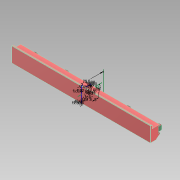
# Autodesk Inventor part: RailVCoverST
Saved by Autodesk Inventor 2021 (Build 250183000, 183)
## iProperties
Created: 2021-03-17
Part Number: RailVCoverST
Material: 一般
Document SubType Name: Modeling
Designer: kumagai
Density: 1 g/cm^3
Appearance: 滑らか - 濃い海緑
Length: 185.000 mm
PrinterOffset: 0.000 mm
StraightLength: 215.000 mm
RailWidth: 38.000 mm
OuterWall: 2.000 mm
InnerWall: 2.400 mm
InsideWidth: 18.600 mm
RailHeight: 8.400 mm
RailDepth: 3.200 mm
ConnectorLength: 15.000 mm
JointMW1: 13.000 mm
JointMW2: 9.400 mm
JointMH: 9.000 mm
JointFW1: 13.300 mm
JointFW2: 9.600 mm
JointFH: 9.500 mm
DoubleWidth: 60.000 mm
ViaductHeight: 66.000 mm
SupportGap: 0.200 mm
SupportRib: 0.500 mm
FixInterval: 41.250 mm
FixNum: 5.000 ul
Author: kumagai
Autodesk Inventor part; units mm, degrees
ref_plane "YZ Plane" through (0, 0, 0) normal (1, 0, 0) x (0, 1, 0)
ref_plane "XZ Plane" through (0, 0, 0) normal (0, 1, 0) x (-1, 0, 0)
ref_plane "XY Plane" through (0, 0, 0) normal (0, 0, 1) x (1, 0, 0)
sketch "スケッチ1" plane through (0, 0, 0) normal (1, 0, 0) x (0, 1, 0)
  line L0 (-5.88, 0) -> (5.88, 0) projected
  line L1 (0, 22.8) -> (0, -3.8) projected
  line L2 (1, 9.3) -> (1, 17)
  line L3 (1, 17) -> (4.2, 17)
  line L4 (4.2, 17) -> (4.2, 19)
  line L5 (4.2, 19) -> (-4.2, 19)
  line L6 (-4.2, 19) -> (-4.2, 17)
  line L7 (-4.2, 17) -> (-1, 17)
  line L8 (-1, 17) -> (-1, 9.3)
  line L9 (-1, 9.3) -> (-4.2, 9.3)
  line L10 (-4.2, 9.3) -> (-4.2, 6.9)
  line L11 (-4.2, 6.9) -> (-1, 6.9)
  line L12 (-1, 6.9) -> (-1, 0)
  line L13 (1, 9.3) -> (4.2, 9.3)
  line L14 (4.2, 9.3) -> (4.2, 6.9)
  line L15 (4.2, 6.9) -> (1, 6.9)
  line L16 (1, 6.9) -> (1, 0)
  line L17 (-4.2, 19) -> (-4.2, 17)
  line L18 (4.2, 17) -> (3.7, 17)
  point P0 (0, 0)
  dimension "d0" = 19
  dimension "d1" = 8.4
  dimension "d2" = 3.2
  dimension "d3" = 2
  dimension "d4" = 2.4
  dimension "d5" = 9.3
  constraints: 34 end point, 13 point on line, 9 perpendicular, 2 collinear, 1 horizontal, 1 vertical, 2 other
  measures "d0" distance between parallel lines of L5 L0
  measures "d1" distance between parallel lines of L6 L4
  measures "d2" distance between parallel lines of L16 L14
  measures "d3" distance between parallel lines of L5 L3
  measures "d4" distance between parallel lines of L15 L13
  measures "d5" distance between parallel lines of L0 L13
sketch "スケッチ2" plane through (0, 0, 0) normal (1, 0, 0) x (0, 1, 0)
  line L0 (10, 29.5) -> (-10, 29.5)
  line L1 (-10, 29.5) -> (-10, 22.3641)
  line L2 (10, 27.5) -> (10, 29.5)
  line L3 (-4.299, 19.1) -> (-4.299, 17)
  line L4 (4.6, 17.1) -> (5.22, 17.1)
  line L5 (4.6, 26.3) -> (3.5931, 27.5)
  line L6 (5.22, 17.1) -> (5.62, 17.5)
  line L7 (5.62, 17.5) -> (5.62, 27.5)
  line L8 (0, 34.06) -> (0, 2.14) projected
  line L9 (-14, 0) -> (14, 0) projected
  line L10 (4.2, 17) -> (4.2, 19) projected
  line L11 (-4.299, 19.1) -> (-4.299, 17)
  line L12 (-5.299, 24.1048) -> (-5.299, 26.3)
  line L13 (-5.299, 26.3) -> (-6.3059, 27.5)
  line L14 (-9.4, 23.2048) -> (-5.299, 23.2048)
  line L15 (-5.299, 23.2048) -> (-5.299, 20)
  line L16 (-9.4, 27.5) -> (-6.3059, 27.5)
  line L17 (-4.299, 27.5) -> (3.5931, 27.5)
  line L18 (5.62, 27.5) -> (10, 27.5)
  line L19 (-5.299, 20) -> (-6.7109, 20)
  line L20 (-10, 22.3641) -> (-5.499, 17)
  line L21 (3.5931, 20.4) -> (-4.299, 20.4)
  line L22 (-9.4, 27.5) -> (-9.4, 24.1048)
  line L23 (-9.4, 23.2048) -> (-6.7109, 20)
  line L24 (-5.299, 24.1048) -> (-9.4, 24.1048)
  line L25 (-4.299, 27.5) -> (-4.299, 20.4)
  line L26 (-4.299, 24.3119) -> (-4.299, 20.4)
  line L27 (4.6, 26.3) -> (4.6, 21.4069)
  line L28 (4.6, 21.4069) -> (3.5931, 20.4)
  line L29 (-4.2, 19) -> (-4.2, 17) projected
  line L30 (4.2, 19) -> (-4.2, 19) projected
  line L31 (-4.299, 17) -> (-5.499, 17)
  line L32 (-4.299, 19.1) -> (4.3, 19.1)
  line L33 (4.3, 19.1) -> (4.6, 18.5804)
  line L34 (4.6, 18.5804) -> (4.6, 17.1)
  line L35 (-1, 9.3) -> (-4.2, 9.3) projected
  line L36 (-4.2, 9.3) -> (-4.2, 6.9) projected
  line L37 (-4.2, 6.9) -> (-1, 6.9) projected
  line L38 (-4.299, 17) -> (-4.299, 6.7)
  line L39 (-4.299, 6.7) -> (-9.299, 6.7)
  line L40 (-9.299, 6.7) -> (-10, 7.5354)
  line L41 (-10, 16.6215) -> (-7.5247, 13.6715)
  line L42 (-7.5247, 13.6715) -> (-6.299, 14.7)
  line L43 (-6.299, 14.7) -> (-10, 19.1107)
  line L44 (-10, 7.5354) -> (-10, 16.6215)
  line L45 (-10, 19.1107) -> (-10, 22.3641)
  point P0 (-3.7, 17)
  point P1 (-3.2, 19)
  point P2 (3.7, 17)
  point P3 (0, 20.4)
  dimension "d63" = 29.5
  dimension "d71" = 2
  dimension "d72" = 40
  dimension "d73" = 1.2
  dimension "d93" = 0.2
  dimension "d109" = 40
  dimension "d110" = 2
  dimension "d113" = 1
  dimension "d114" = 0.6
  dimension "d115" = 0.9
  dimension "d117" = 1
  dimension "d128" = 1.02
  dimension "d129" = 45
  dimension "d130" = 0.4
  dimension "d141" = 0.099
  dimension "d142" = 5.8
  dimension "d143" = 5.8
  dimension "d144" = 3
  dimension "d145" = 0.1
  dimension "d146" = 1.3
  dimension "d147" = 30
  dimension "d148" = 0.1
  dimension "d149" = 0.4
  dimension "d150" = 0.1
  dimension "d151" = 45
  dimension "d152" = 0.2
  dimension "d153" = 5
  dimension "d156" = 1.6
  dimension "d157" = 2
  dimension "d158" = 8
  constraints: 77 end point, 16 perpendicular, 9 parallel, 6 horizontal, 5 collinear, 5 vertical, 3 point on line, 1 horizontal alignment, 1 vertical alignment
  measures "d63" distance between parallel lines of L0 L9
  measures "d71" distance between parallel lines of L0 L16
  measures "d72" angle of L12 L13
  measures "d73" distance from line of L12.end L16
  measures "d93" horizontal distance of L20.end L15.end
  measures "d109" angle of L8 L20
  measures "d110" distance between parallel lines of L0 L18
  measures "d113" distance between parallel lines of L20 L23
  measures "d114" distance between parallel lines of L1 L22
  measures "d115" distance between parallel lines of L24 L14
  measures "d117" distance between parallel lines of L12 L26
  measures "d128" distance between parallel lines of L7 L27
  measures "d129" angle of L4 L6
  measures "d130" distance from line of L4 L6.end
  measures "d141" distance between parallel lines of L3 L29
  measures "d142" distance between parallel lines of L1 L29
  measures "d143" distance between parallel lines of L2 L10
  measures "d144" distance between parallel lines of L31 L19
  measures "d145" distance between parallel lines of L30 L32
  measures "d146" distance between parallel lines of L21 L32
  measures "d147" angle of L10 L33
  measures "d148" distance from line of L10 L32.end
  measures "d149" distance between parallel lines of L10 L34
  measures "d150" distance from line of L4 L10.start
  measures "d151" angle of L27 L28
  measures "d152" distance between parallel lines of L39 L37
  measures "d153" distance from line of L39.end L38
  measures "d156" distance between parallel lines of L41 L43
  measures "d157" distance from line of L38 L42.end
  measures "d158" distance from line of L39 L42.end
extrude "押し出し3" [suppressed]
extrude "押し出し4" add sketch "スケッチ2" along normal mid plane 185 contours L2 L18 L7 L6 L4 L34 L33 L32 L8 L21 L28 L27 L5 L17 L0 | L8 L17 L25 L21 L32 L3 L31 L20 L1 L0
chamfer "面取り1" distance 0.4 angle 45 2 edges at (0, 10, 29.5) (0, 10, 27.5)
sketch "スケッチ3" plane through (92.5, 0, 0) normal (1, 0, 0) x (0, 0, -1)
  line L0 (-27.9, 10) -> (-27.5, 9.6) projected
  line L1 (-27.9, 10) -> (-29.1, 10) projected
  line L2 (-29.5, 9.6) -> (-29.1, 10) projected
  line L3 (-29.5, 9.6) -> (-29.5, -10) projected
  line L4 (-29.5, -10) -> (-22.3641, -10) projected
  line L5 (-22.3641, -10) -> (-17, -5.499) projected
  line L6 (-17, -4.299) -> (-19.1, -4.299) projected
  line L7 (-17.1, 4.6) -> (-17.1, 5.22) projected
  line L8 (-17.1, 5.22) -> (-17.5, 5.62) projected
  line L9 (-17.5, 5.62) -> (-27.5, 5.62) projected
  line L10 (-27.5, 5.62) -> (-27.5, 9.6) projected
  line L11 (-27.5, -9.4) -> (-27.5, -6.3059) projected
  line L12 (-27.5, -6.3059) -> (-26.3, -5.299) projected
  line L13 (-26.3, -5.299) -> (-24.1048, -5.299) projected
  line L14 (-24.1048, -5.299) -> (-24.1048, -9.4) projected
  line L15 (-24.1048, -9.4) -> (-27.5, -9.4) projected
  line L16 (-23.2048, -9.4) -> (-23.2048, -5.299) projected
  line L17 (-23.2048, -5.299) -> (-20, -5.299) projected
  line L18 (-20, -5.299) -> (-20, -6.7109) projected
  line L19 (-20, -6.7109) -> (-23.2048, -9.4) projected
  line L20 (-26.3, 4.6) -> (-21.4069, 4.6) projected
  line L21 (-21.4069, 4.6) -> (-20.4, 3.5931) projected
  line L22 (-20.4, 3.5931) -> (-20.4, -4.299) projected
  line L23 (-20.4, -4.299) -> (-27.5, -4.299) projected
  line L24 (-27.5, -4.299) -> (-27.5, 3.5931) projected
  line L25 (-27.5, 3.5931) -> (-26.3, 4.6) projected
  line L26 (-17, -5.499) -> (-17, -4.299) projected
  line L27 (-19.1, -4.299) -> (-19.1, 4.3) projected
  line L28 (-19.1, 4.3) -> (-18.5804, 4.6) projected
  line L29 (-18.5804, 4.6) -> (-17.1, 4.6) projected
  point P0 (0, 0)
extrude "押し出し5" add sketch "スケッチ3" against normal blind 1 contours L11 L12 L13 L14 L15 | L16 L17 L18 L19 | L20 L21 L22 L23 L24 L25
sketch "スケッチ5" plane through (-92.5, 0, 0) normal (-1, 0, 0) x (0, 0, 1)
  line L0 (27.5, 9.6) -> (27.9, 10) projected
  line L1 (27.5, 9.6) -> (27.5, 5.62) projected
  line L2 (27.5, 5.62) -> (17.5, 5.62) projected
  line L3 (17.5, 5.62) -> (17.1, 5.22) projected
  line L4 (17.1, 5.22) -> (17.1, 4.6) projected
  line L5 (19.1, -4.299) -> (17, -4.299) projected
  line L6 (17, -5.499) -> (22.3641, -10) projected
  line L7 (22.3641, -10) -> (29.5, -10) projected
  line L8 (29.5, -10) -> (29.5, 9.6) projected
  line L9 (29.1, 10) -> (29.5, 9.6) projected
  line L10 (29.1, 10) -> (27.9, 10) projected
  line L11 (27.5, -6.3059) -> (27.5, -9.4) projected
  line L12 (27.5, -9.4) -> (24.1048, -9.4) projected
  line L13 (24.1048, -9.4) -> (24.1048, -5.299) projected
  line L14 (24.1048, -5.299) -> (26.3, -5.299) projected
  line L15 (26.3, -5.299) -> (27.5, -6.3059) projected
  line L16 (23.2048, -5.299) -> (23.2048, -9.4) projected
  line L17 (23.2048, -9.4) -> (20, -6.7109) projected
  line L18 (20, -6.7109) -> (20, -5.299) projected
  line L19 (20, -5.299) -> (23.2048, -5.299) projected
  line L20 (21.4069, 4.6) -> (26.3, 4.6) projected
  line L21 (26.3, 4.6) -> (27.5, 3.5931) projected
  line L22 (27.5, 3.5931) -> (27.5, -4.299) projected
  line L23 (27.5, -4.299) -> (20.4, -4.299) projected
  line L24 (20.4, -4.299) -> (20.4, 3.5931) projected
  line L25 (20.4, 3.5931) -> (21.4069, 4.6) projected
  line L26 (17.1, 4.6) -> (18.5804, 4.6) projected
  line L27 (18.5804, 4.6) -> (19.1, 4.3) projected
  line L28 (19.1, 4.3) -> (19.1, -4.299) projected
  line L29 (17, -4.299) -> (17, -5.499) projected
  point P0 (0, 0)
extrude "押し出し6" add sketch "スケッチ5" against normal blind 1 contours L11 L12 L13 L14 L15 | L16 L17 L18 L19 | L20 L21 L22 L23 L24 L25
chamfer "面取り2" distance 0.4 angle 45 8 edges at (92.5, 10, 28.5) (92.5, -0.2, 29.5) (92.5, -10, 25.932) (92.5, -7.7495, 19.682) (-92.5, 10, 28.5) (-92.5, -0.2, 29.5) (-92.5, -10, 25.932) (-92.5, -7.7495, 19.682)
extrude "押し出し7" add sketch "スケッチ2" along normal mid plane 4 contours L20 L31 L38 L39 L40 L44 L41 L42 L43 L45
chamfer "面取り3" distance 0.4 angle 45 6 edges at (2, -8.1495, 16.9053) (2, -6.9118, 14.1858) (2, -8.7623, 15.1465) (-2, -8.7623, 15.1465) (-2, -6.9118, 14.1858) (-2, -8.1495, 16.9053)
pattern_linear "矩形状パターン1" count 5 spacing 41.25 along (1, 0, 0) of "押し出し7", "面取り3" first direction both ways yes
equation "\"d0\" = 0.5 * RailWidth"
equation "\"d2\" = RailDepth"
equation "\"d4\" = InnerWall"
equation "\"d5\" = 0.5 * InsideWidth"
equation "\"d101\" = SupportRib"
equation "\"Length\" = 185"
equation "\"FixInterval\" = 41.25"
equation "\"FixNum\" = 5"
equation "\"RailWidth\" = 38"
equation "\"RailDepth\" = 3.2"
equation "\"InnerWall\" = 2.4"
equation "\"InsideWidth\" = 18.6"
equation "\"SupportRib\" = 0.5"
